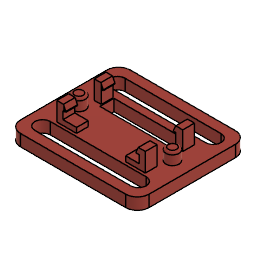
LaserDistanceSensor (Autodesk Fusion 360 design; units mm, degrees)
Autodesk Fusion 360 part; units mm, degrees
sketch "Sketch1" plane through (0, 0, 0) normal (0, 0, 1) x (1, 0, 0)
  line L0 (0, 0) -> (15.5, 0)
  line L1 (15.5, 10.5) -> (0, 10.5)
  circle A0 centre (-2.5, 5.25) radius 1.5
  line L2 (-2.5, 7.75) -> (0, 7.75)
  line L3 (-2.5, 2.75) -> (0, 2.75)
  arc A1 (-2.5, 7.75) -> (-2.5, 2.75) centre (-2.5, 5.25) ccw
  line L4 (0, 10.5) -> (0, 7.75)
  line L5 (0, 2.75) -> (0, 0)
  line L6 (7.75, 10.5) -> (7.75, 0) construction
  line L7 (18, 2.75) -> (15.5, 2.75)
  line L8 (18, 7.75) -> (15.5, 7.75)
  circle A2 centre (18, 5.25) radius 1.5
  arc A3 (18, 2.75) -> (18, 7.75) centre (18, 5.25) ccw
  line L9 (15.5, 0) -> (15.5, 2.75)
  line L10 (15.5, 7.75) -> (15.5, 10.5)
  dimension "d1" = 15.5
  dimension "d2" = 10.5
  dimension "d4" = 3
  dimension "d5" = 5
  constraint horizontal L0
  constraint vertical L9
  constraint horizontal L1
  constraint vertical L4
  constraint coincident L0.start L5.end
  constraint tangent L2 A1
  constraint perpendicular L2 L4
  constraint tangent L3 A1
  constraint collinear L4 L5
  constraint midpoint L1 L6.start
  constraint midpoint L0 L6.end
  constraint symmetric A0 L6 A2
  constraint symmetric L2.start L6 L8.start
  constraint symmetric L2.end L6 L8.end
  constraint symmetric L3.start L6 L7.start
  constraint symmetric L3.end L6 L7.end
  constraint symmetric A1 L6 A3
  constraint collinear L9 L10
  measures "d1" distance of L0.start L0.end
  measures "d2" distance of L0.start L1.end
  measures "d4" diameter of A0
  measures "d5" diameter of A1
extrude "Extrude1" add sketch "Sketch1" along normal blind 1.2 makes body 1
sketch "Sketch2" plane through (0, 0, 1.2) normal (0, 0, 1) x (-1, 0, 0)
  circle A0 centre (-18, -5.25) radius 1.5
  circle A1 centre (2.5, -5.25) radius 1.5
  arc A2 (-18, -2.75) -> (-18, -7.75) centre (-18, -5.25) ccw
  line L0 (-18, -7.75) -> (-15.5, -7.75)
  line L1 (-15.5, -7.75) -> (-15.5, -10.5)
  line L2 (-15.5, -10.5) -> (0, -10.5)
  line L3 (0, -10.5) -> (0, -7.75)
  line L4 (0, -7.75) -> (2.5, -7.75)
  arc A3 (2.5, -7.75) -> (2.5, -2.75) centre (2.5, -5.25) ccw
  line L5 (2.5, -2.75) -> (0, -2.75)
  line L6 (0, -2.75) -> (0, 0)
  line L7 (0, 0) -> (-15.5, 0)
  line L8 (-15.5, 0) -> (-15.5, -2.75)
  line L9 (-15.5, -2.75) -> (-18, -2.75)
  line L10 (0, 0) -> (-0.25, 0)
  line L11 (-0.25, 0) -> (-0.25, -0.25)
  line L12 (-0.25, -0.25) -> (-15.25, -0.25)
  line L13 (-15.25, -0.25) -> (-15.25, -2.75)
  line L14 (-15.25, -2.75) -> (-0.25, -2.75)
  line L15 (-0.25, -2.75) -> (-0.25, -0.25)
  line L16 (-0.25, -2.75) -> (-2.75, -2.75) construction
  circle A4 centre (-2.75, -2.75) radius 0.05
  circle A5 centre (-5.25, -2.75) radius 0.05
  circle A6 centre (-7.75, -2.75) radius 0.05
  circle A7 centre (-10.25, -2.75) radius 0.05
  circle A8 centre (-12.75, -2.75) radius 0.05
  circle A9 centre (-2.75, -0.25) radius 0.05
  circle A10 centre (-5.25, -0.25) radius 0.05
  circle A11 centre (-7.75, -0.25) radius 0.05
  circle A12 centre (-10.25, -0.25) radius 0.05
  circle A13 centre (-12.75, -0.25) radius 0.05
  circle A14 centre (-0.25, -2.75) radius 0.05
  circle A15 centre (-0.25, -0.25) radius 0.05
  circle A16 centre (-15.25, -2.75) radius 0.05
  circle A17 centre (-15.25, -0.25) radius 0.05
  dimension "d8" = 0.25
  dimension "d9" = 0.25
  dimension "d10" = 15
  dimension "d11" = 2.5
  dimension "d12" = 2.5
  dimension "d13" = 0.1
  dimension "d16" = -10
  dimension "d17" = 2.5
  dimension "d20" = 0.1
  dimension "d21" = 0.1
  dimension "d22" = 0.1
  dimension "d23" = 0.1
  constraint coincident L6.end L7.start
  constraint coincident L7 L10.end
  constraint perpendicular L7 L11
  constraint horizontal L12
  constraint vertical L13
  constraint horizontal L14
  constraint vertical L15
  constraint perpendicular L15 L16
  constraint coincident L16.end A4.centre
  constraint coincident L14.end L15.start
  constraint coincident L11.end L12.start
  constraint coincident L13.end L14.start
  constraint coincident L12.end L13.start
  measures "d8" distance of L6.end L10.end
  measures "d9" distance of L10.end L11.end
  measures "d10" distance of L11.end L12.end
  measures "d11" distance of L11.end L14.end
  measures "d12" distance of L14.end L16.end
  measures "d13" diameter of A4
  measures "d20" diameter of A14
  measures "d21" diameter of A15
  measures "d22" diameter of A16
  measures "d23" diameter of A17
extrude "Extrude2" add sketch "Sketch2" along normal blind 2.5 contours L12 L13 L14 L15 A4 A5 A6 A7 A8 A9 A10 A11 A12 A13 A14 A15 A16 A17 bodies 1
sketch "Sketch3" plane through (0, 0, 0) normal (0, 0, -1) x (1, 0, 0)
  circle A0 centre (18, -5.25) radius 1.5
  circle A1 centre (-2.5, -5.25) radius 1.5
  arc A2 (18, -7.75) -> (18, -2.75) centre (18, -5.25) ccw
  line L0 (18, -2.75) -> (15.5, -2.75)
  line L1 (15.5, -2.75) -> (15.5, 0)
  line L2 (15.5, 0) -> (0, 0)
  line L3 (0, 0) -> (0, -2.75)
  line L4 (0, -2.75) -> (-2.5, -2.75)
  arc A3 (-2.5, -2.75) -> (-2.5, -7.75) centre (-2.5, -5.25) ccw
  line L5 (-2.5, -7.75) -> (0, -7.75)
  line L6 (0, -7.75) -> (0, -10.5)
  line L7 (0, -10.5) -> (15.5, -10.5)
  line L8 (15.5, -10.5) -> (15.5, -7.75)
  line L9 (15.5, -7.75) -> (18, -7.75)
  line L10 (0, -2.75) -> (0, -0.25) construction
  line L11 (0, -1.375) -> (1.5, -1.375) construction
  circle A4 centre (1.5, -1.375) radius 0.75
  circle A5 centre (4, -1.375) radius 0.75
  circle A6 centre (6.5, -1.375) radius 0.75
  circle A7 centre (9, -1.375) radius 0.75
  circle A8 centre (11.5, -1.375) radius 0.75
  circle A9 centre (14, -1.375) radius 0.75
  line L12 (7.75, -10.5) -> (7.75, -9) construction
  line L13 (7.75, -9) -> (9.95, -9)
  line L14 (9.95, -9) -> (9.95, -7.8)
  line L15 (9.95, -9) -> (5.55, -9)
  line L16 (5.55, -9) -> (5.55, -6.6)
  line L17 (5.55, -6.6) -> (9.95, -6.6)
  line L18 (9.95, -6.6) -> (9.95, -9)
  dimension "d24" = 2.5
  dimension "d25" = 1.5
  dimension "d26" = 1.5
  dimension "d29" = 12.5
  dimension "d30" = 0
  dimension "d31" = 1.5
  dimension "d32" = 2.2
  dimension "d34" = 4.4
  dimension "d35" = 2.4
  constraint coincident L3.end L4.start
  constraint coincident L3 L10.end
  constraint midpoint L3 L11.start
  constraint perpendicular L3 L11
  constraint coincident L11.end A4.centre
  constraint midpoint L7 L12.start
  constraint perpendicular L7 L12
  constraint horizontal L13
  constraint vertical L14
  constraint horizontal L15
  constraint vertical L16
  constraint horizontal L17
  constraint vertical L18
  measures "d24" distance of L3.end L10.end
  measures "d25" distance of L11.start L11.end
  measures "d26" diameter of A4
  measures "d31" distance of L12.start L12.end
  measures "d32" distance of L12.end L13.end
  measures "d34" distance of L13.end L15.end
  measures "d35" distance of L13.end L17.end
extrude "Extrude3" add sketch "Sketch3" along normal blind 1 draft -30 contours A4 | A5 | A6 | A7 | A8 | A9 bodies 1
extrude "Extrude4" add sketch "Sketch3" along normal blind 1 contours L13 L14 L15 L16 L17 L18 bodies 1
sketch "Sketch4" plane through (0, 0, 1.2) normal (0, 0, 1) x (-1, 0, 0)
  arc A0 (-10.3, -0.25) -> (-10.2, -0.25) centre (-10.25, -0.25) ccw
  line L0 (-10.2, -0.25) -> (-7.8, -0.25)
  arc A1 (-7.8, -0.25) -> (-7.7, -0.25) centre (-7.75, -0.25) ccw
  line L1 (-7.7, -0.25) -> (-5.3, -0.25)
  arc A2 (-5.3, -0.25) -> (-5.2, -0.25) centre (-5.25, -0.25) ccw
  line L2 (-5.2, -0.25) -> (-2.8, -0.25)
  arc A3 (-2.8, -0.25) -> (-2.7, -0.25) centre (-2.75, -0.25) ccw
  line L3 (-2.7, -0.25) -> (-0.3, -0.25)
  arc A4 (-0.3, -0.25) -> (-0.25, -0.3) centre (-0.25, -0.25) ccw
  line L4 (-0.25, -0.3) -> (-0.25, -2.7)
  arc A5 (-0.25, -2.7) -> (-0.3, -2.75) centre (-0.25, -2.75) ccw
  line L5 (-0.3, -2.75) -> (-2.7, -2.75)
  arc A6 (-2.7, -2.75) -> (-2.8, -2.75) centre (-2.75, -2.75) ccw
  line L6 (-2.8, -2.75) -> (-5.2, -2.75)
  arc A7 (-5.2, -2.75) -> (-5.3, -2.75) centre (-5.25, -2.75) ccw
  line L7 (-5.3, -2.75) -> (-7.7, -2.75)
  arc A8 (-7.7, -2.75) -> (-7.8, -2.75) centre (-7.75, -2.75) ccw
  line L8 (-7.8, -2.75) -> (-10.2, -2.75)
  arc A9 (-10.2, -2.75) -> (-10.3, -2.75) centre (-10.25, -2.75) ccw
  line L9 (-10.3, -2.75) -> (-12.7, -2.75)
  arc A10 (-12.7, -2.75) -> (-12.8, -2.75) centre (-12.75, -2.75) ccw
  line L10 (-12.8, -2.75) -> (-15.2, -2.75)
  arc A11 (-15.2, -2.75) -> (-15.25, -2.7) centre (-15.25, -2.75) ccw
  line L11 (-15.25, -2.7) -> (-15.25, -0.3)
  arc A12 (-15.25, -0.3) -> (-15.2, -0.25) centre (-15.25, -0.25) ccw
  line L12 (-15.2, -0.25) -> (-12.8, -0.25)
  arc A13 (-12.8, -0.25) -> (-12.7, -0.25) centre (-12.75, -0.25) ccw
  line L13 (-12.7, -0.25) -> (-10.3, -0.25)
  circle A14 centre (-18, -5.25) radius 1.5
  circle A15 centre (2.5, -5.25) radius 1.5
  arc A16 (-18, -2.75) -> (-18, -7.75) centre (-18, -5.25) ccw
  line L14 (-18, -7.75) -> (-15.5, -7.75)
  line L15 (-15.5, -7.75) -> (-15.5, -10.5)
  line L16 (-15.5, -10.5) -> (0, -10.5)
  line L17 (0, -10.5) -> (0, -7.75)
  line L18 (0, -7.75) -> (2.5, -7.75)
  arc A17 (2.5, -7.75) -> (2.5, -2.75) centre (2.5, -5.25) ccw
  line L19 (2.5, -2.75) -> (0, -2.75)
  line L20 (0, -2.75) -> (0, 0)
  line L21 (0, 0) -> (-15.5, 0)
  line L22 (-15.5, 0) -> (-15.5, -2.75)
  line L23 (-15.5, -2.75) -> (-18, -2.75)
  line L24 (-10, -8.5) -> (-9, -8.5)
  line L25 (-9, -8.5) -> (-9, -10)
  line L26 (-9, -10) -> (-10, -10)
  line L27 (-10, -10) -> (-10, -8.5)
  line L28 (-8.5, -8.5) -> (-7.5, -8.5)
  line L29 (-7.5, -8.5) -> (-7.5, -10)
  line L30 (-7.5, -10) -> (-8.5, -10)
  line L31 (-8.5, -10) -> (-8.5, -8.5)
  line L32 (-7, -8.5) -> (-6, -8.5)
  line L33 (-6, -8.5) -> (-6, -10)
  line L34 (-6, -10) -> (-7, -10)
  line L35 (-7, -10) -> (-7, -8.5)
  line L36 (-2.5, -4.5) -> (-1.5, -4.5)
  line L37 (-3, -4.5) -> (-3, -6)
  line L38 (-4, -4.5) -> (-3, -4.5)
  line L39 (-3, -6) -> (-4, -6)
  line L40 (-2.5, -6) -> (-2.5, -4.5)
  line L41 (-4, -6) -> (-4, -4.5)
  line L42 (-1.5, -4.5) -> (-1.5, -6)
  line L43 (-1.5, -6) -> (-2.5, -6)
  line L44 (-10.5, -3.5) -> (-9, -3.5)
  line L45 (-9, -3.5) -> (-9, -8)
  line L46 (-9, -8) -> (-10.5, -8)
  line L47 (-10.5, -8) -> (-10.5, -3.5)
  line L48 (-7.5, -4) -> (-5.5, -4)
  line L49 (-5.5, -4) -> (-5.5, -5.5)
  line L50 (-5.5, -5.5) -> (-7.5, -5.5)
  line L51 (-7.5, -5.5) -> (-7.5, -4)
  line L52 (-14.5, -3.5) -> (-13, -3.5)
  line L53 (-13, -3.5) -> (-13, -4.5)
  line L54 (-13, -4.5) -> (-14.5, -4.5)
  line L55 (-14.5, -4.5) -> (-14.5, -3.5)
  line L56 (-14.5, -5.5) -> (-11.5, -5.5)
  line L57 (-11.5, -5.5) -> (-11.5, -7)
  line L58 (-11.5, -7) -> (-14.5, -7)
  line L59 (-14.5, -7) -> (-14.5, -5.5)
  dimension "d40" = 1.5
  constraint horizontal L24
  constraint vertical L25
  constraint horizontal L26
  constraint vertical L27
  constraint horizontal L28
  constraint vertical L29
  constraint horizontal L30
  constraint vertical L31
  constraint horizontal L32
  constraint vertical L33
  constraint horizontal L34
  constraint vertical L35
  constraint horizontal L38
  constraint vertical L37
  constraint horizontal L39
  constraint vertical L41
  constraint horizontal L36
  constraint vertical L42
  constraint horizontal L43
  constraint vertical L40
  constraint horizontal L44
  constraint vertical L45
  constraint horizontal L46
  constraint vertical L47
  constraint horizontal L48
  constraint vertical L49
  constraint horizontal L50
  constraint vertical L51
  constraint horizontal L52
  constraint vertical L53
  constraint horizontal L54
  constraint vertical L55
  constraint horizontal L56
  constraint vertical L57
  constraint horizontal L58
  constraint vertical L59
  measures "d40" distance of L48.start L50.end
extrude "Extrude5" add sketch "Sketch4" along normal blind 1 contours L24 L25 L26 L27 | L28 L29 L30 L31 | L32 L33 L34 L35 | L36 L40 L42 L43 | L37 L38 L39 L41 | L44 L45 L46 L47 | L48 L49 L50 L51 | L52 L53 L54 L55 | L56 L57 L58 L59 bodies 1
sketch "Sketch5" plane through (0, 0, 3.7) normal (0, 0, 1) x (-1, 0, 0)
  line L0 (-10.3, -0.25) -> (-12.7, -0.25)
  arc A0 (-12.8, -0.25) -> (-12.7, -0.25) centre (-12.75, -0.25) ccw
  line L1 (-12.8, -0.25) -> (-15.2, -0.25)
  arc A1 (-15.25, -0.3) -> (-15.2, -0.25) centre (-15.25, -0.25) ccw
  line L2 (-15.25, -0.3) -> (-15.25, -2.7)
  arc A2 (-15.2, -2.75) -> (-15.25, -2.7) centre (-15.25, -2.75) ccw
  line L3 (-15.2, -2.75) -> (-12.8, -2.75)
  arc A3 (-12.7, -2.75) -> (-12.8, -2.75) centre (-12.75, -2.75) ccw
  line L4 (-12.7, -2.75) -> (-10.3, -2.75)
  arc A4 (-10.2, -2.75) -> (-10.3, -2.75) centre (-10.25, -2.75) ccw
  line L5 (-10.2, -2.75) -> (-7.8, -2.75)
  arc A5 (-7.7, -2.75) -> (-7.8, -2.75) centre (-7.75, -2.75) ccw
  line L6 (-7.7, -2.75) -> (-5.3, -2.75)
  arc A6 (-5.2, -2.75) -> (-5.3, -2.75) centre (-5.25, -2.75) ccw
  line L7 (-5.2, -2.75) -> (-2.8, -2.75)
  arc A7 (-2.7, -2.75) -> (-2.8, -2.75) centre (-2.75, -2.75) ccw
  line L8 (-2.7, -2.75) -> (-0.3, -2.75)
  arc A8 (-0.25, -2.7) -> (-0.3, -2.75) centre (-0.25, -2.75) ccw
  line L9 (-0.25, -2.7) -> (-0.25, -0.3)
  arc A9 (-0.3, -0.25) -> (-0.25, -0.3) centre (-0.25, -0.25) ccw
  line L10 (-0.3, -0.25) -> (-2.7, -0.25)
  arc A10 (-2.8, -0.25) -> (-2.7, -0.25) centre (-2.75, -0.25) ccw
  line L11 (-2.8, -0.25) -> (-5.2, -0.25)
  arc A11 (-5.3, -0.25) -> (-5.2, -0.25) centre (-5.25, -0.25) ccw
  line L12 (-5.3, -0.25) -> (-7.7, -0.25)
  arc A12 (-7.8, -0.25) -> (-7.7, -0.25) centre (-7.75, -0.25) ccw
  line L13 (-7.8, -0.25) -> (-10.2, -0.25)
  arc A13 (-10.3, -0.25) -> (-10.2, -0.25) centre (-10.25, -0.25) ccw
  line L14 (-0.25, -1.5) -> (-1.5, -1.5) construction
  line L15 (-1.25, -1.25) -> (-1.75, -1.25)
  line L16 (-1.75, -1.25) -> (-1.75, -1.75)
  line L17 (-1.75, -1.75) -> (-1.25, -1.75)
  line L18 (-1.25, -1.75) -> (-1.25, -1.25)
  line L19 (-1.25, -1.25) -> (-1.75, -1.75) construction
  line L20 (-1.75, -1.25) -> (-1.25, -1.75) construction
  line L21 (-4.25, -1.75) -> (-3.75, -1.75)
  line L22 (-3.75, -1.75) -> (-3.75, -1.25)
  line L23 (-3.75, -1.25) -> (-4.25, -1.25)
  line L24 (-4.25, -1.25) -> (-4.25, -1.75)
  line L25 (-6.75, -1.75) -> (-6.25, -1.75)
  line L26 (-6.25, -1.75) -> (-6.25, -1.25)
  line L27 (-6.25, -1.25) -> (-6.75, -1.25)
  line L28 (-6.75, -1.25) -> (-6.75, -1.75)
  line L29 (-9.25, -1.75) -> (-8.75, -1.75)
  line L30 (-8.75, -1.75) -> (-8.75, -1.25)
  line L31 (-8.75, -1.25) -> (-9.25, -1.25)
  line L32 (-9.25, -1.25) -> (-9.25, -1.75)
  line L33 (-11.75, -1.75) -> (-11.25, -1.75)
  line L34 (-11.25, -1.75) -> (-11.25, -1.25)
  line L35 (-11.25, -1.25) -> (-11.75, -1.25)
  line L36 (-11.75, -1.25) -> (-11.75, -1.75)
  line L37 (-14.25, -1.75) -> (-13.75, -1.75)
  line L38 (-13.75, -1.75) -> (-13.75, -1.25)
  line L39 (-13.75, -1.25) -> (-14.25, -1.25)
  line L40 (-14.25, -1.25) -> (-14.25, -1.75)
  point P0 (-1.5, -1.5)
  dimension "d43" = 0.5
  dimension "d44" = 0.5
  dimension "d47" = -12.5
  dimension "d48" = 0
  constraint midpoint L9 L14.start
  constraint perpendicular L9 L14
  constraint horizontal L15
  constraint perpendicular L15 L16
  constraint parallel L15 L17
  constraint parallel L16 L18
  constraint coincident L19 P0
  constraint coincident L20 P0
  constraint coincident P0 L14.end
  measures "d43" distance of L16.end L17.end
  measures "d44" distance of L15.end L16.end
extrude "Extrude6" add sketch "Sketch5" along normal blind 5 contours L15 L16 L17 L18 | L21 L22 L23 L24 | L25 L26 L27 L28 | L29 L30 L31 L32 | L33 L34 L35 L36 | L37 L38 L39 L40 bodies 1
sketch "Sketch6" plane through (0, 0, 0) normal (0, 0, 1) x (1, 0, 0)
  line L0 (0, 10.5) -> (15.5, 10.5) construction
  line L1 (15.5, 10.5) -> (15.5, 0) construction
  line L2 (15.5, 0) -> (0, 0) construction
  line L3 (0, 0) -> (0, 10.5) construction
  line L4 (0, 8) -> (-5, 8) construction
  line L5 (-5, 8) -> (-5, 2.5) construction
  line L6 (-5, 2.5) -> (0, 2.5) construction
  line L7 (0, 2.5) -> (0, 8) construction
  line L8 (20.5, 8) -> (15.5, 8) construction
  line L9 (15.5, 8) -> (15.5, 2.5) construction
  line L10 (15.5, 2.5) -> (20.5, 2.5) construction
  line L11 (20.5, 2.5) -> (20.5, 8) construction
  line L12 (-2.5, 5.25) -> (-2.5, 13.25) construction
  line L13 (-2.5, 13.25) -> (-2.5, -2.75) construction
  line L14 (18, 5.25) -> (18, -2.75) construction
  line L15 (17.9885, -4.4) -> (-2.5, -4.4)
  line L16 (18, -1.1) -> (-2.5, -1.1)
  line L17 (18, 11.6) -> (-2.5, 11.6)
  line L18 (-2.5, 14.9) -> (18, 14.9)
  arc A0 (-2.5, 14.9) -> (-2.5, 11.6) centre (-2.5, 13.25) ccw
  arc A1 (18, 11.6) -> (18, 14.9) centre (18, 13.25) ccw
  arc A2 (17.9885, -4.4) -> (18, -1.1) centre (18, -2.75) ccw
  arc A3 (-2.5, -1.1) -> (-2.5, -4.4) centre (-2.5, -2.75) ccw
  line L19 (-2.5, 13.25) -> (-2.5, 17) construction
  line L20 (-2.5, 17) -> (-6, 17) construction
  line L21 (-3.5, 17) -> (19, 17)
  line L22 (21.5, 14.5) -> (21.5, -4)
  line L23 (19, -6.5) -> (-3.5, -6.5)
  line L24 (-6, -4) -> (-6, 14.5)
  arc A4 (-3.5, 17) -> (-6, 14.5) centre (-3.5, 14.5) ccw
  arc A5 (-6, -4) -> (-3.5, -6.5) centre (-3.5, -4) ccw
  arc A6 (19, -6.5) -> (21.5, -4) centre (19, -4) ccw
  arc A7 (21.5, 14.5) -> (19, 17) centre (19, 14.5) ccw
  dimension "d51" = 8
  dimension "d52" = 16
  dimension "d53" = 3.3
  dimension "d54" = 3.3
  dimension "d55" = 8
  dimension "d56" = 3.3
  dimension "d57" = 3.3
  dimension "d58" = 2.5
  constraint horizontal L0
  constraint vertical L1
  constraint horizontal L2
  constraint vertical L3
  constraint horizontal L4
  constraint vertical L5
  constraint horizontal L6
  constraint vertical L7
  constraint coincident L3 L4.start
  constraint horizontal L8
  constraint vertical L9
  constraint horizontal L10
  constraint vertical L11
  constraint coincident L1 L9.end
  constraint perpendicular L4 L12
  constraint perpendicular L6 L13
  constraint coincident L12.end L13.start
  constraint coincident L13.end A3.centre
  constraint perpendicular L10 L14
  constraint coincident L14.end A2.centre
  constraint tangent L15 A3
  constraint coincident L14 L16.start
  constraint coincident L13 L16.end
  constraint tangent L16 A3
  constraint coincident L13 L17.end
  constraint tangent L18 A1
  constraint parallel L17 L18
  constraint perpendicular L18 L19
  constraint perpendicular L19 L20
  constraint horizontal L21
  constraint vertical L22
  constraint horizontal L23
  constraint vertical L24
  constraint coincident L20.end L21
  constraint coincident L20.end L24
  constraint tangent L21 A4
  constraint tangent L24 A4
  constraint tangent L23 A5
  constraint tangent L24 A5
  constraint equal A4 A5
  constraint tangent L22 A6
  constraint tangent L23 A6
  constraint equal A4 A6
  constraint tangent L21 A7
  constraint tangent L22 A7
  constraint equal A4 A7
  measures "d51" distance of L12.start L12.end
  measures "d52" distance of L12.end L13.end
  measures "d53" diameter of A0
  measures "d54" diameter of A3
  measures "d55" distance of L14.start L14.end
  measures "d56" diameter of A2
  measures "d57" diameter of A1
  measures "d58" radius of A4
extrude "Extrude7" add sketch "Sketch6" against normal blind 2.5 separate body makes body 2
move_body "Move1" bodies 1 to x (1, 0, 0) y (0, 1, 0) z (0, 0, 1) at (0, 0.5, -5)
sketch "Sketch7" plane through (0, 0, -2.5) normal (0, 0, -1) x (1, 0, 0)
  arc A0 (-2.5, -11.6) -> (-2.5, -14.9) centre (-2.5, -13.25) ccw
  line L0 (-2.5, -11.6) -> (18, -11.6)
  arc A1 (18, -14.9) -> (18, -11.6) centre (18, -13.25) ccw
  line L1 (18, -14.9) -> (-2.5, -14.9)
  arc A2 (18, 1.1) -> (17.9885, 4.4) centre (18, 2.75) ccw
  line L2 (18, 1.1) -> (-2.5, 1.1)
  arc A3 (-2.5, 4.4) -> (-2.5, 1.1) centre (-2.5, 2.75) ccw
  line L3 (-2.5, 4.4) -> (17.9885, 4.4)
  arc A4 (21.5, 4) -> (19, 6.5) centre (19, 4) ccw
  line L4 (19, 6.5) -> (-3.5, 6.5)
  arc A5 (-3.5, 6.5) -> (-6, 4) centre (-3.5, 4) ccw
  line L5 (-6, 4) -> (-6, -14.5)
  arc A6 (-6, -14.5) -> (-3.5, -17) centre (-3.5, -14.5) ccw
  line L6 (-3.5, -17) -> (19, -17)
  arc A7 (19, -17) -> (21.5, -14.5) centre (19, -14.5) ccw
  line L7 (21.5, -14.5) -> (21.5, 4)
  line L8 (15.7, -11) -> (17.2, -11)
  line L9 (17.2, -11) -> (17.2, -8.5)
  line L10 (17.2, -8.5) -> (15.7, -8.5)
  line L11 (15.7, -8.5) -> (15.7, -11)
  line L12 (-1.7, -11) -> (-0.2, -11)
  line L13 (-0.2, -11) -> (-0.2, -8.5)
  line L14 (-0.2, -8.5) -> (-1.7, -8.5)
  line L15 (-1.7, -8.5) -> (-1.7, -11)
  circle A8 centre (17.75, -5.75) radius 1.4
  line L16 (-0.2, -11) -> (2.5, -11)
  line L17 (2.5, -11) -> (2.5, -8.5)
  line L18 (2.5, -8.5) -> (-0.2, -8.5)
  line L19 (-0.2, -8.5) -> (-0.2, -11)
  line L20 (15.7, -8.5) -> (13, -8.5)
  line L21 (13, -8.5) -> (13, -11)
  line L22 (13, -11) -> (15.7, -11)
  line L23 (15.7, -11) -> (15.7, -8.5)
  circle A9 centre (-2.25, -5.75) radius 1.4
  line L24 (15.5, -0.5) -> (0, -0.5)
  line L25 (0, -0.5) -> (0, -3.5)
  line L26 (0, -3.5) -> (15.5, -3.5)
  line L27 (15.5, -3.5) -> (15.5, -0.5)
  dimension "d61" = 2.8
  dimension "d62" = 2.8
  dimension "d99" = 10.5
  constraint horizontal L8
  constraint vertical L9
  constraint horizontal L10
  constraint vertical L11
  constraint horizontal L12
  constraint vertical L13
  constraint horizontal L14
  constraint vertical L15
  constraint horizontal L16
  constraint vertical L17
  constraint horizontal L18
  constraint vertical L19
  constraint horizontal L20
  constraint vertical L21
  constraint horizontal L22
  constraint vertical L23
  constraint horizontal L24
  constraint vertical L25
  constraint horizontal L26
  constraint vertical L27
  measures "d61" diameter of A8
  measures "d62" diameter of A9
  measures "d99" distance of L17 L21
extrude "Extrude8" cut sketch "Sketch7" against normal blind 5 contours L24 L25 L26 L27 bodies 2
extrude "Extrude9" add sketch "Sketch7" along normal blind 1.5 contours L11 L20 L21 L22 L23 | L13 L16 L17 L18 L19 bodies 2
move_body "Move2" bodies 1 to x (1, 0, 0) y (0, 1, 0) z (0, 0, 1) at (0, 0, -0.3)
extrude "Extrude10" add sketch "Sketch7" along normal blind 4 contours L8 L9 L10 L11 L23 | L12 L13 L14 L15 L19 | A8 | A9 bodies 2
sketch "Sketch8" plane through (0, 0, -6.5) normal (0, 0, -1) x (1, 0, 0)
  line L0 (-1.7, -8.5) -> (-1.7, -11)
  line L1 (-1.7, -11) -> (-0.2, -11)
  line L2 (-0.2, -11) -> (-0.2, -8.5)
  line L3 (-0.2, -8.5) -> (-1.7, -8.5)
  line L4 (-0.2, -8.5) -> (0.2, -8.5)
  line L5 (0.2, -8.5) -> (0.2, -11.0027)
  line L6 (0.2, -11.0027) -> (-0.2, -11.0027)
  line L7 (-0.2, -11.0027) -> (-0.2, -8.5)
  line L8 (15.7, -8.5) -> (15.2, -8.5)
  line L9 (15.2, -8.5) -> (15.2, -11)
  line L10 (15.2, -11) -> (15.7, -11)
  line L11 (15.7, -11) -> (15.7, -8.5)
  dimension "d84" = 0.4
  dimension "d85" = 0.5
  constraint horizontal L4
  constraint vertical L5
  constraint horizontal L6
  constraint vertical L7
  constraint coincident L2.end L3.start
  constraint horizontal L8
  constraint vertical L9
  constraint horizontal L10
  constraint vertical L11
  measures "d84" distance of L5 L7
  measures "d85" distance of L9 L11
extrude "Extrude11" add sketch "Sketch8" against normal blind 1.25 contours L2 L4 L5 L6 L7 | L8 L9 L10 L11 bodies 2
chamfer "Chamfer1" distance 1.1 distance2 0.5 1 edges at (0.2, 9.7513, -6.5) measured on face at (0.2, 9.3342, -6.0833) on bodies 2
chamfer "Chamfer2" distance 0.5 distance2 1.1 1 edges at (15.2, 9.75, -6.5) measured on face at (15.8667, 9.3333, -6.5) on bodies 2
extrude "Extrude12" cut 2 faces at (0.7, 9.3333, -4) (14.8, 10.1667, -4) along direction (0, 0, 1) blind 0.2 on bodies 2 bodies 2
extrude "Extrude15" cut 1 faces at (-0.2, 10.1667, -4.7667) along direction (-1, 0, 0) blind 0.1 on bodies 2 bodies 2
extrude "Extrude16" cut 1 faces at (15.7, 9.3333, -4.7667) along direction (1, 0, 0) blind 0.1 on bodies 2 bodies 2
extrude "Extrude21" cut 2 faces at (-2.8993, 5.2846, -6.5) (17.5129, 5.295, -6.5) along direction (0, 0, 1) blind 1.5 on bodies 2 bodies 2
fillet "Fillet1" radius 0.5 2 edges at (16.4447, 5.2437, -5) (-3.5553, 5.2437, -5) on bodies 2
extrude "Extrude17" cut 2 faces at (14.8667, 10.1667, -3.8) (0.6333, 9.3333, -3.8) along direction (0, 0, 1) blind 0.1 on bodies 2 bodies 2
extrude "Extrude18" cut 2 faces at (14.8667, 10.1667, -3.7) (0.6333, 9.3333, -3.7) along direction (0, 0, 1) blind 0.1 on bodies 2 bodies 2
extrude "Extrude19" cut 1 faces at (15.8, 9.3333, -4.7667) along direction (1, 0, 0) blind 0.1 on bodies 2 bodies 2
extrude "Extrude20" cut 1 faces at (-0.3, 10.1667, -4.7) along direction (-1, 0, 0) blind 0.1 on bodies 2 bodies 2
pattern_linear "R-Pattern1" count 2 spacing 8 along (0, -1, 0) of "Extrude10", "Extrude11", "Chamfer1", "Chamfer2"
extrude "Extrude22" cut 2 faces at (17.5129, -2.705, -6.5) (-2.8993, -2.7154, -6.5) along direction (0, 0, 1) blind 4 on bodies 2 bodies 2
move_body "Move3" bodies 2 to x (1, 0, 0) y (0, -1, 0) z (0, 0, -1) at (0, 10.5, 0)
hidden bodies 1
equation "d25 = 0.25 mm + 1.25 mm"
named bodies: "DistanceSenzorHolder"
